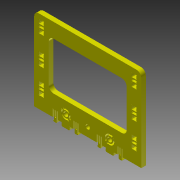
# Autodesk Inventor part: back
Saved by Autodesk Inventor 2012 (Build 160160000, 160)
## iProperties
Created: 2011-10-14
Part Number: back
Document SubType Name: Modeling
Designer: cramera
Density: 0.952 g/cm^3
Material: High Density Polyethylene
Mass: 370.231 g
Surface Area: 1050.09 cm^2
Volume: 388.898 cm^3
Autodesk Inventor part; units mm, degrees
ref_plane "YZ Plane" through (0, 0, 0) normal (1, 0, 0) x (0, 1, 0)
ref_plane "XZ Plane" through (0, 0, 0) normal (0, 1, 0) x (-1, 0, 0)
ref_plane "XY Plane" through (0, 0, 0) normal (0, 0, 1) x (1, 0, 0)
derived "skeleton.ipt"
sketch "POCKET_1-16" plane through (0, 0, 0) normal (0, 0, 1) x (1, 0, 0)
  circle A0 centre (662.3461, 379.1269) radius 7.3978
  constraints: 1 centre point
sketch "STOCK_12MM" plane through (0, 0, 0) normal (0, 0, 1) x (1, 0, 0)
  line L0 (457.2, 914.4) -> (457.2, 0)
  line L1 (457.2, 0) -> (457.2, 914.4)
  line L2 (457.2, 0) -> (914.4, 0)
  line L3 (914.4, 0) -> (914.4, 914.4)
  line L4 (914.4, 914.4) -> (457.2, 914.4)
  constraints: 10 end point
sketch "THROUGH-CUT" plane through (0, 0, 0) normal (0, 0, 1) x (1, 0, 0)
  arc A0 (777.0271, 478.4952) -> (779.2722, 476.2502) centre (778.1496, 477.3727) ccw
  line L0 (777.0271, 478.4952) -> (777.0271, 484.1651)
  arc A1 (779.2722, 486.4102) -> (777.0271, 484.1651) centre (778.1496, 485.2876) ccw
  line L1 (779.2722, 486.4102) -> (787.101, 486.4102)
  arc A2 (789.3461, 486.4102) -> (787.101, 486.4102) centre (788.2236, 485.2876) ccw
  arc A3 (789.3461, 484.1651) -> (789.3461, 486.4102) centre (788.2236, 485.2876) ccw
  line L2 (789.3461, 484.1651) -> (789.3461, 478.4952)
  arc A4 (789.3461, 476.2502) -> (789.3461, 478.4952) centre (788.2236, 477.3727) ccw
  arc A5 (787.101, 476.2502) -> (789.3461, 476.2502) centre (788.2236, 477.3727) ccw
  line L3 (787.101, 476.2502) -> (779.2722, 476.2502)
  line L4 (777.0271, 403.4382) -> (777.0271, 404.0281)
  arc A6 (777.0271, 406.2732) -> (777.0271, 404.0281) centre (778.1496, 405.1506) ccw
  arc A7 (779.2722, 406.2732) -> (777.0271, 406.2732) centre (778.1496, 405.1506) ccw
  line L5 (779.2722, 406.2732) -> (787.101, 406.2732)
  arc A8 (789.3461, 406.2732) -> (787.101, 406.2732) centre (788.2236, 405.1506) ccw
  arc A9 (789.3461, 404.0281) -> (789.3461, 406.2732) centre (788.2236, 405.1506) ccw
  line L6 (789.3461, 404.0281) -> (789.3461, 403.4382)
  arc A10 (787.101, 401.1932) -> (789.3461, 403.4382) centre (788.2236, 402.3157) ccw
  line L7 (787.101, 401.1932) -> (779.2722, 401.1932)
  arc A11 (777.0271, 403.4382) -> (779.2722, 401.1932) centre (778.1496, 402.3157) ccw
  line L8 (547.6651, 543.7281) -> (547.6651, 543.1382)
  arc A12 (547.6651, 540.8932) -> (547.6651, 543.1382) centre (546.5426, 542.0157) ccw
  arc A13 (545.42, 540.8932) -> (547.6651, 540.8932) centre (546.5426, 542.0157) ccw
  line L9 (545.42, 540.8932) -> (537.5912, 540.8932)
  arc A14 (535.3461, 543.1382) -> (537.5912, 540.8932) centre (536.4686, 542.0157) ccw
  line L10 (535.3461, 543.1382) -> (535.3461, 543.7281)
  arc A15 (535.3461, 545.9732) -> (535.3461, 543.7281) centre (536.4686, 544.8506) ccw
  arc A16 (537.5912, 545.9732) -> (535.3461, 545.9732) centre (536.4686, 544.8506) ccw
  line L11 (537.5912, 545.9732) -> (545.42, 545.9732)
  arc A17 (547.6651, 543.7281) -> (545.42, 545.9732) centre (546.5426, 544.8506) ccw
  circle A18 centre (719.4961, 379.1269) radius 5.925
  circle A19 centre (605.1961, 379.1269) radius 5.925
  circle A20 centre (662.3461, 379.1269) radius 5.5563
  line L12 (547.6651, 395.6461) -> (547.6651, 389.9762)
  arc A21 (547.6651, 387.7312) -> (547.6651, 389.9762) centre (546.5426, 388.8537) ccw
  arc A22 (545.42, 387.7312) -> (547.6651, 387.7312) centre (546.5426, 388.8537) ccw
  line L13 (545.42, 387.7312) -> (537.5912, 387.7312)
  arc A23 (535.3461, 389.9762) -> (537.5912, 387.7312) centre (536.4686, 388.8537) ccw
  line L14 (535.3461, 389.9762) -> (535.3461, 395.6461)
  arc A24 (537.5912, 397.8912) -> (535.3461, 395.6461) centre (536.4686, 396.7686) ccw
  line L15 (537.5912, 397.8912) -> (545.42, 397.8912)
  arc A25 (547.6651, 395.6461) -> (545.42, 397.8912) centre (546.5426, 396.7686) ccw
  line L16 (777.0271, 529.6762) -> (777.0271, 535.3461)
  arc A26 (777.0271, 537.5912) -> (777.0271, 535.3461) centre (778.1496, 536.4686) ccw
  arc A27 (779.2722, 537.5912) -> (777.0271, 537.5912) centre (778.1496, 536.4686) ccw
  line L17 (779.2722, 537.5912) -> (787.101, 537.5912)
  arc A28 (789.3461, 537.5912) -> (787.101, 537.5912) centre (788.2236, 536.4686) ccw
  arc A29 (789.3461, 535.3461) -> (789.3461, 537.5912) centre (788.2236, 536.4686) ccw
  line L18 (789.3461, 535.3461) -> (789.3461, 529.6762)
  arc A30 (789.3461, 527.4312) -> (789.3461, 529.6762) centre (788.2236, 528.5537) ccw
  arc A31 (787.101, 527.4312) -> (789.3461, 527.4312) centre (788.2236, 528.5537) ccw
  line L19 (787.101, 527.4312) -> (779.2722, 527.4312)
  arc A32 (777.0271, 529.6762) -> (779.2722, 527.4312) centre (778.1496, 528.5537) ccw
  line L20 (547.6651, 404.0281) -> (547.6651, 403.4382)
  arc A33 (547.6651, 401.1932) -> (547.6651, 403.4382) centre (546.5426, 402.3157) ccw
  arc A34 (545.42, 401.1932) -> (547.6651, 401.1932) centre (546.5426, 402.3157) ccw
  line L21 (545.42, 401.1932) -> (537.5912, 401.1932)
  arc A35 (535.3461, 403.4382) -> (537.5912, 401.1932) centre (536.4686, 402.3157) ccw
  line L22 (535.3461, 403.4382) -> (535.3461, 404.0281)
  arc A36 (537.5912, 406.2732) -> (535.3461, 404.0281) centre (536.4686, 405.1506) ccw
  line L23 (537.5912, 406.2732) -> (545.42, 406.2732)
  arc A37 (547.6651, 406.2732) -> (545.42, 406.2732) centre (546.5426, 405.1506) ccw
  arc A38 (547.6651, 404.0281) -> (547.6651, 406.2732) centre (546.5426, 405.1506) ccw
  line L24 (779.2722, 559.4352) -> (787.101, 559.4352)
  arc A39 (789.3461, 559.4352) -> (787.101, 559.4352) centre (788.2236, 558.3126) ccw
  arc A40 (789.3461, 557.1901) -> (789.3461, 559.4352) centre (788.2236, 558.3126) ccw
  line L25 (789.3461, 557.1901) -> (789.3461, 551.5202)
  arc A41 (789.3461, 549.2752) -> (789.3461, 551.5202) centre (788.2236, 550.3977) ccw
  arc A42 (787.101, 549.2752) -> (789.3461, 549.2752) centre (788.2236, 550.3977) ccw
  line L26 (787.101, 549.2752) -> (779.2722, 549.2752)
  arc A43 (777.0271, 549.2752) -> (779.2722, 549.2752) centre (778.1496, 550.3977) ccw
  arc A44 (777.0271, 551.5202) -> (777.0271, 549.2752) centre (778.1496, 550.3977) ccw
  line L27 (777.0271, 551.5202) -> (777.0271, 557.1901)
  arc A45 (779.2722, 559.4352) -> (777.0271, 557.1901) centre (778.1496, 558.3126) ccw
  arc A46 (779.2722, 419.7352) -> (777.0271, 417.4901) centre (778.1496, 418.6126) ccw
  line L28 (779.2722, 419.7352) -> (787.101, 419.7352)
  arc A47 (789.3461, 419.7352) -> (787.101, 419.7352) centre (788.2236, 418.6126) ccw
  arc A48 (789.3461, 417.4901) -> (789.3461, 419.7352) centre (788.2236, 418.6126) ccw
  line L29 (789.3461, 417.4901) -> (789.3461, 411.8202)
  arc A49 (789.3461, 409.5752) -> (789.3461, 411.8202) centre (788.2236, 410.6977) ccw
  arc A50 (787.101, 409.5752) -> (789.3461, 409.5752) centre (788.2236, 410.6977) ccw
  line L30 (787.101, 409.5752) -> (779.2722, 409.5752)
  arc A51 (777.0271, 411.8202) -> (779.2722, 409.5752) centre (778.1496, 410.6977) ccw
  line L31 (777.0271, 411.8202) -> (777.0271, 417.4901)
  arc A52 (777.0271, 456.6512) -> (779.2722, 454.4062) centre (778.1496, 455.5287) ccw
  line L32 (777.0271, 456.6512) -> (777.0271, 462.3211)
  arc A53 (779.2722, 464.5662) -> (777.0271, 462.3211) centre (778.1496, 463.4436) ccw
  line L33 (779.2722, 464.5662) -> (787.101, 464.5662)
  arc A54 (789.3461, 464.5662) -> (787.101, 464.5662) centre (788.2236, 463.4436) ccw
  arc A55 (789.3461, 462.3211) -> (789.3461, 464.5662) centre (788.2236, 463.4436) ccw
  line L34 (789.3461, 462.3211) -> (789.3461, 456.6512)
  arc A56 (789.3461, 454.4062) -> (789.3461, 456.6512) centre (788.2236, 455.5287) ccw
  arc A57 (787.101, 454.4062) -> (789.3461, 454.4062) centre (788.2236, 455.5287) ccw
  line L35 (787.101, 454.4062) -> (779.2722, 454.4062)
  arc A58 (777.0271, 389.9762) -> (777.0271, 387.7312) centre (778.1496, 388.8537) ccw
  line L36 (777.0271, 389.9762) -> (777.0271, 395.6461)
  arc A59 (779.2722, 397.8912) -> (777.0271, 395.6461) centre (778.1496, 396.7686) ccw
  line L37 (779.2722, 397.8912) -> (787.101, 397.8912)
  arc A60 (789.3461, 397.8912) -> (787.101, 397.8912) centre (788.2236, 396.7686) ccw
  arc A61 (789.3461, 395.6461) -> (789.3461, 397.8912) centre (788.2236, 396.7686) ccw
  line L38 (789.3461, 395.6461) -> (789.3461, 389.9762)
  arc A62 (787.101, 387.7312) -> (789.3461, 389.9762) centre (788.2236, 388.8537) ccw
  line L39 (787.101, 387.7312) -> (779.2722, 387.7312)
  arc A63 (777.0271, 387.7312) -> (779.2722, 387.7312) centre (778.1496, 388.8537) ccw
  line L40 (547.6651, 484.1651) -> (547.6651, 478.4952)
  arc A64 (547.6651, 476.2502) -> (547.6651, 478.4952) centre (546.5426, 477.3727) ccw
  arc A65 (545.42, 476.2502) -> (547.6651, 476.2502) centre (546.5426, 477.3727) ccw
  line L41 (545.42, 476.2502) -> (537.5912, 476.2502)
  arc A66 (535.3461, 478.4952) -> (537.5912, 476.2502) centre (536.4686, 477.3727) ccw
  line L42 (535.3461, 478.4952) -> (535.3461, 484.1651)
  arc A67 (537.5912, 486.4102) -> (535.3461, 484.1651) centre (536.4686, 485.2876) ccw
  line L43 (537.5912, 486.4102) -> (545.42, 486.4102)
  arc A68 (547.6651, 484.1651) -> (545.42, 486.4102) centre (546.5426, 485.2876) ccw
  arc A69 (777.0271, 543.1382) -> (777.0271, 540.8932) centre (778.1496, 542.0157) ccw
  line L44 (777.0271, 543.1382) -> (777.0271, 543.7281)
  arc A70 (779.2722, 545.9732) -> (777.0271, 543.7281) centre (778.1496, 544.8506) ccw
  line L45 (779.2722, 545.9732) -> (787.101, 545.9732)
  arc A71 (789.3461, 545.9732) -> (787.101, 545.9732) centre (788.2236, 544.8506) ccw
  arc A72 (789.3461, 543.7281) -> (789.3461, 545.9732) centre (788.2236, 544.8506) ccw
  line L46 (789.3461, 543.7281) -> (789.3461, 543.1382)
  arc A73 (789.3461, 540.8932) -> (789.3461, 543.1382) centre (788.2236, 542.0157) ccw
  arc A74 (787.101, 540.8932) -> (789.3461, 540.8932) centre (788.2236, 542.0157) ccw
  line L47 (787.101, 540.8932) -> (779.2722, 540.8932)
  arc A75 (777.0271, 540.8932) -> (779.2722, 540.8932) centre (778.1496, 542.0157) ccw
  line L48 (547.6651, 470.7031) -> (547.6651, 470.1132)
  arc A76 (547.6651, 467.8682) -> (547.6651, 470.1132) centre (546.5426, 468.9907) ccw
  arc A77 (545.42, 467.8682) -> (547.6651, 467.8682) centre (546.5426, 468.9907) ccw
  line L49 (545.42, 467.8682) -> (537.5912, 467.8682)
  arc A78 (535.3461, 470.1132) -> (537.5912, 467.8682) centre (536.4686, 468.9907) ccw
  line L50 (535.3461, 470.1132) -> (535.3461, 470.7031)
  arc A79 (537.5912, 472.9482) -> (535.3461, 470.7031) centre (536.4686, 471.8256) ccw
  line L51 (537.5912, 472.9482) -> (545.42, 472.9482)
  arc A80 (547.6651, 470.7031) -> (545.42, 472.9482) centre (546.5426, 471.8256) ccw
  line L52 (547.6651, 417.4901) -> (547.6651, 411.8202)
  arc A81 (547.6651, 409.5752) -> (547.6651, 411.8202) centre (546.5426, 410.6977) ccw
  arc A82 (545.42, 409.5752) -> (547.6651, 409.5752) centre (546.5426, 410.6977) ccw
  line L53 (545.42, 409.5752) -> (537.5912, 409.5752)
  arc A83 (535.3461, 411.8202) -> (537.5912, 409.5752) centre (536.4686, 410.6977) ccw
  line L54 (535.3461, 411.8202) -> (535.3461, 417.4901)
  arc A84 (537.5912, 419.7352) -> (535.3461, 417.4901) centre (536.4686, 418.6126) ccw
  line L55 (537.5912, 419.7352) -> (545.42, 419.7352)
  arc A85 (547.6651, 417.4901) -> (545.42, 419.7352) centre (546.5426, 418.6126) ccw
  line L56 (547.6651, 557.1901) -> (547.6651, 551.5202)
  arc A86 (547.6651, 549.2752) -> (547.6651, 551.5202) centre (546.5426, 550.3977) ccw
  arc A87 (545.42, 549.2752) -> (547.6651, 549.2752) centre (546.5426, 550.3977) ccw
  line L57 (545.42, 549.2752) -> (537.5912, 549.2752)
  arc A88 (535.3461, 551.5202) -> (537.5912, 549.2752) centre (536.4686, 550.3977) ccw
  line L58 (535.3461, 551.5202) -> (535.3461, 557.1901)
  arc A89 (537.5912, 559.4352) -> (535.3461, 557.1901) centre (536.4686, 558.3126) ccw
  line L59 (537.5912, 559.4352) -> (545.42, 559.4352)
  arc A90 (547.6651, 557.1901) -> (545.42, 559.4352) centre (546.5426, 558.3126) ccw
  line L60 (535.3461, 456.6512) -> (535.3461, 462.3211)
  arc A91 (537.5912, 464.5662) -> (535.3461, 462.3211) centre (536.4686, 463.4436) ccw
  line L61 (537.5912, 464.5662) -> (545.42, 464.5662)
  arc A92 (547.6651, 462.3211) -> (545.42, 464.5662) centre (546.5426, 463.4436) ccw
  line L62 (547.6651, 462.3211) -> (547.6651, 456.6512)
  arc A93 (545.42, 454.4062) -> (547.6651, 456.6512) centre (546.5426, 455.5287) ccw
  line L63 (545.42, 454.4062) -> (537.5912, 454.4062)
  arc A94 (535.3461, 456.6512) -> (537.5912, 454.4062) centre (536.4686, 455.5287) ccw
  arc A95 (777.0271, 470.1132) -> (777.0271, 467.8682) centre (778.1496, 468.9907) ccw
  line L64 (777.0271, 470.1132) -> (777.0271, 470.7031)
  arc A96 (779.2722, 472.9482) -> (777.0271, 470.7031) centre (778.1496, 471.8256) ccw
  line L65 (779.2722, 472.9482) -> (787.101, 472.9482)
  arc A97 (789.3461, 472.9482) -> (787.101, 472.9482) centre (788.2236, 471.8256) ccw
  arc A98 (789.3461, 470.7031) -> (789.3461, 472.9482) centre (788.2236, 471.8256) ccw
  line L66 (789.3461, 470.7031) -> (789.3461, 470.1132)
  arc A99 (787.101, 467.8682) -> (789.3461, 470.1132) centre (788.2236, 468.9907) ccw
  line L67 (787.101, 467.8682) -> (779.2722, 467.8682)
  arc A100 (777.0271, 467.8682) -> (779.2722, 467.8682) centre (778.1496, 468.9907) ccw
  line L68 (535.3461, 529.6762) -> (535.3461, 535.3461)
  arc A101 (537.5912, 537.5912) -> (535.3461, 535.3461) centre (536.4686, 536.4686) ccw
  line L69 (537.5912, 537.5912) -> (545.42, 537.5912)
  arc A102 (547.6651, 535.3461) -> (545.42, 537.5912) centre (546.5426, 536.4686) ccw
  line L70 (547.6651, 535.3461) -> (547.6651, 529.6762)
  arc A103 (545.42, 527.4312) -> (547.6651, 529.6762) centre (546.5426, 528.5537) ccw
  line L71 (545.42, 527.4312) -> (537.5912, 527.4312)
  arc A104 (535.3461, 529.6762) -> (537.5912, 527.4312) centre (536.4686, 528.5537) ccw
  arc A105 (723.7603, 390.4675) -> (708.1555, 374.8628) centre (719.4961, 379.1269) ccw
  line L72 (708.1555, 374.8628) -> (707.4839, 374.1911)
  arc A106 (707.4839, 374.1911) -> (707.4839, 371.9461) centre (708.6064, 373.0686) ccw
  line L73 (707.4839, 371.9461) -> (707.5557, 371.8742)
  arc A107 (707.5557, 371.8742) -> (709.8008, 371.8742) centre (708.6782, 372.9968) ccw
  line L74 (709.8008, 371.8742) -> (711.2845, 373.3579)
  arc A108 (711.2845, 373.3579) -> (711.5831, 375.1879) centre (710.1619, 374.4805) ccw
  arc A109 (723.4351, 387.0399) -> (711.5831, 375.1879) centre (719.4961, 379.1269) ccw
  arc A110 (723.4351, 387.0399) -> (725.2651, 387.3385) centre (724.1426, 388.4611) ccw
  line L75 (725.2651, 387.3385) -> (726.7488, 388.8223)
  arc A111 (726.7488, 388.8223) -> (726.7488, 391.0673) centre (725.6263, 389.9448) ccw
  line L76 (726.7488, 391.0673) -> (726.677, 391.1392)
  arc A112 (726.677, 391.1392) -> (724.4319, 391.1392) centre (725.5544, 390.0166) ccw
  line L77 (724.4319, 391.1392) -> (723.7603, 390.4675)
  line L78 (763.9461, 521.2082) -> (763.9461, 422.7832)
  arc A113 (751.2461, 410.0832) -> (763.9461, 422.7832) centre (751.2461, 422.7832) ccw
  line L79 (751.2461, 410.0832) -> (573.4461, 410.0832)
  arc A114 (560.7461, 422.7832) -> (573.4461, 410.0832) centre (573.4461, 422.7832) ccw
  line L80 (560.7461, 422.7832) -> (560.7461, 521.2082)
  arc A115 (573.4461, 533.9082) -> (560.7461, 521.2082) centre (573.4461, 521.2082) ccw
  line L81 (573.4461, 533.9082) -> (751.2461, 533.9082)
  arc A116 (763.9461, 521.2082) -> (751.2461, 533.9082) centre (751.2461, 521.2082) ccw
  arc A117 (577.9048, 357.2797) -> (579.4923, 358.8672) centre (577.9048, 358.8672) ccw
  line L82 (577.9048, 357.2797) -> (577.7778, 357.2797)
  arc A118 (576.1903, 358.8672) -> (577.7778, 357.2797) centre (577.7778, 358.8672) ccw
  line L83 (576.1903, 358.8672) -> (576.1903, 373.5707)
  arc A119 (577.7778, 375.1582) -> (576.1903, 373.5707) centre (577.7778, 373.5707) ccw
  line L84 (577.7778, 375.1582) -> (577.9048, 375.1582)
  arc A120 (579.4923, 373.5707) -> (577.9048, 375.1582) centre (577.9048, 373.5707) ccw
  line L85 (579.4923, 373.5707) -> (579.4923, 358.8672)
  arc A121 (692.6854, 357.2797) -> (694.2729, 358.8672) centre (692.6854, 358.8672) ccw
  line L86 (692.6854, 357.2797) -> (692.5584, 357.2797)
  arc A122 (690.9709, 358.8672) -> (692.5584, 357.2797) centre (692.5584, 358.8672) ccw
  line L87 (690.9709, 358.8672) -> (690.9709, 373.5707)
  arc A123 (692.5584, 375.1582) -> (690.9709, 373.5707) centre (692.5584, 373.5707) ccw
  line L88 (692.5584, 375.1582) -> (692.6732, 375.1582)
  arc A124 (694.2607, 373.5707) -> (692.6732, 375.1582) centre (692.6732, 373.5707) ccw
  line L89 (694.2607, 373.5707) -> (694.2729, 358.8672)
  arc A125 (745.1999, 358.8672) -> (746.7874, 357.2797) centre (746.7874, 358.8672) ccw
  line L90 (746.7874, 357.2797) -> (746.9144, 357.2797)
  arc A126 (746.9144, 357.2797) -> (748.5019, 358.8672) centre (746.9144, 358.8672) ccw
  line L91 (748.5019, 358.8672) -> (748.5019, 373.5707)
  arc A127 (748.5019, 373.5707) -> (746.9144, 375.1582) centre (746.9144, 373.5707) ccw
  line L92 (746.9144, 375.1582) -> (746.7874, 375.1582)
  arc A128 (746.7874, 375.1582) -> (745.1999, 373.5707) centre (746.7874, 373.5707) ccw
  line L93 (745.1999, 373.5707) -> (745.1999, 358.8672)
  arc A129 (632.1338, 357.2797) -> (633.7213, 358.8672) centre (632.1338, 358.8672) ccw
  line L94 (633.7213, 358.8672) -> (633.7213, 373.5707)
  arc A130 (633.7213, 373.5707) -> (632.1338, 375.1582) centre (632.1338, 373.5707) ccw
  line L95 (632.1338, 375.1582) -> (632.0068, 375.1582)
  arc A131 (632.0068, 375.1582) -> (630.4193, 373.5707) centre (632.0068, 373.5707) ccw
  line L96 (630.4193, 373.5707) -> (630.4193, 358.8672)
  arc A132 (630.4193, 358.8672) -> (632.0068, 357.2797) centre (632.0068, 358.8672) ccw
  line L97 (632.0068, 357.2797) -> (632.1338, 357.2797)
  arc A133 (593.1839, 386.3078) -> (593.1839, 384.0627) centre (594.3064, 385.1853) ccw
  line L98 (593.1839, 384.0627) -> (593.8555, 383.3911)
  arc A134 (593.8555, 383.3911) -> (609.4603, 367.7863) centre (605.1961, 379.1269) ccw
  line L99 (609.4603, 367.7863) -> (610.1319, 367.1147)
  arc A135 (610.1319, 367.1147) -> (612.377, 367.1147) centre (611.2544, 368.2372) ccw
  line L100 (612.377, 367.1147) -> (612.4488, 367.1865)
  arc A136 (612.4488, 367.1865) -> (612.4488, 369.4316) centre (611.3263, 368.3091) ccw
  line L101 (612.4488, 369.4316) -> (610.9651, 370.9153)
  arc A137 (610.9651, 370.9153) -> (609.1351, 371.2139) centre (609.8426, 369.7928) ccw
  arc A138 (597.2831, 383.0659) -> (609.1351, 371.2139) centre (605.1961, 379.1269) ccw
  arc A139 (597.2831, 383.0659) -> (596.9845, 384.8959) centre (595.8619, 383.7734) ccw
  line L102 (596.9845, 384.8959) -> (595.5008, 386.3796)
  arc A140 (595.5008, 386.3796) -> (593.2557, 386.3796) centre (594.3782, 385.2571) ccw
  line L103 (593.2557, 386.3796) -> (593.1839, 386.3078)
  arc A141 (617.2083, 371.9461) -> (617.2083, 374.1911) centre (616.0858, 373.0686) ccw
  line L104 (617.2083, 374.1911) -> (616.5367, 374.8628)
  arc A142 (616.5367, 374.8628) -> (600.9319, 390.4675) centre (605.1961, 379.1269) ccw
  line L105 (600.9319, 390.4675) -> (600.2603, 391.1392)
  arc A143 (600.2603, 391.1392) -> (598.0152, 391.1392) centre (599.1378, 390.0166) ccw
  line L106 (598.0152, 391.1392) -> (597.9434, 391.0673)
  arc A144 (597.9434, 391.0673) -> (597.9434, 388.8223) centre (599.0659, 389.9448) ccw
  line L107 (597.9434, 388.8223) -> (599.4271, 387.3385)
  arc A145 (599.4271, 387.3385) -> (601.2571, 387.0399) centre (600.5496, 388.4611) ccw
  arc A146 (613.1091, 375.1879) -> (601.2571, 387.0399) centre (605.1961, 379.1269) ccw
  arc A147 (613.1091, 375.1879) -> (613.4077, 373.3579) centre (614.5302, 374.4805) ccw
  line L108 (613.4077, 373.3579) -> (614.8914, 371.8742)
  arc A148 (614.8914, 371.8742) -> (617.1365, 371.8742) centre (616.014, 372.9968) ccw
  line L109 (617.1365, 371.8742) -> (617.2083, 371.9461)
  line L110 (629.9748, 347.2182) -> (633.6777, 347.2182)
  line L111 (633.6777, 347.2182) -> (637.2773, 348.0403)
  line L112 (637.2773, 348.0403) -> (637.2773, 349.7582)
  line L113 (637.2773, 349.7582) -> (635.7533, 351.0282)
  line L114 (635.7533, 351.0282) -> (635.7533, 353.6554)
  line L115 (635.7533, 353.6554) -> (635.7533, 373.5707)
  arc A149 (637.3408, 375.1582) -> (635.7533, 373.5707) centre (637.3408, 373.5707) ccw
  line L116 (637.3408, 375.1582) -> (637.4678, 375.1582)
  arc A150 (639.0553, 373.5707) -> (637.4678, 375.1582) centre (637.4678, 373.5707) ccw
  line L117 (639.0553, 373.5707) -> (639.0553, 356.1082)
  line L118 (639.0553, 356.1082) -> (685.6369, 356.1082)
  line L119 (685.6369, 356.1082) -> (685.6369, 373.5707)
  arc A151 (687.2244, 375.1582) -> (685.6369, 373.5707) centre (687.2244, 373.5707) ccw
  line L120 (687.2244, 375.1582) -> (687.3514, 375.1582)
  arc A152 (688.9389, 373.5707) -> (687.3514, 375.1582) centre (687.3514, 373.5707) ccw
  line L121 (688.9389, 373.5707) -> (688.9389, 353.6554)
  line L122 (688.9389, 353.6554) -> (688.9389, 351.0282)
  line L123 (688.9389, 351.0282) -> (687.4149, 349.7582)
  line L124 (687.4149, 349.7582) -> (687.4149, 348.0403)
  line L125 (687.4149, 348.0403) -> (691.0145, 347.2182)
  line L126 (691.0145, 347.2182) -> (694.7174, 347.2182)
  arc A153 (694.7174, 347.2182) -> (696.3049, 348.8057) centre (694.7174, 348.8057) ccw
  line L127 (696.3049, 348.8057) -> (696.3049, 373.5707)
  arc A154 (697.8924, 375.1582) -> (696.3049, 373.5707) centre (697.8924, 373.5707) ccw
  line L128 (697.8924, 375.1582) -> (698.0194, 375.1582)
  arc A155 (699.6069, 373.5707) -> (698.0194, 375.1582) centre (698.0194, 373.5707) ccw
  line L129 (699.6069, 373.5707) -> (699.6069, 356.1082)
  line L130 (699.6069, 356.1082) -> (707.0139, 356.1082)
  arc A156 (709.2589, 353.8631) -> (707.0139, 356.1082) centre (708.1364, 354.9856) ccw
  line L131 (709.2589, 353.8631) -> (709.2589, 348.8057)
  line L132 (709.2589, 348.8057) -> (710.8464, 347.2182)
  line L133 (710.8464, 347.2182) -> (728.6264, 347.2182)
  line L134 (728.6264, 347.2182) -> (730.2139, 348.8057)
  line L135 (730.2139, 348.8057) -> (730.2139, 353.8631)
  arc A157 (732.459, 356.1082) -> (730.2139, 353.8631) centre (731.3364, 354.9856) ccw
  line L136 (732.459, 356.1082) -> (739.8659, 356.1082)
  line L137 (739.8659, 356.1082) -> (739.8659, 373.5707)
  arc A158 (741.4534, 375.1582) -> (739.8659, 373.5707) centre (741.4534, 373.5707) ccw
  line L138 (741.4534, 375.1582) -> (741.5804, 375.1582)
  arc A159 (743.1679, 373.5707) -> (741.5804, 375.1582) centre (741.5804, 373.5707) ccw
  line L139 (743.1679, 373.5707) -> (743.1679, 348.8057)
  arc A160 (743.1679, 348.8057) -> (744.7532, 347.2182) centre (744.7554, 348.8057) ccw
  line L140 (744.7532, 347.2182) -> (748.4584, 347.2182)
  line L141 (748.4584, 347.2182) -> (752.0579, 348.0403)
  line L142 (752.0579, 348.0403) -> (752.0579, 349.7582)
  line L143 (752.0579, 349.7582) -> (750.5339, 351.0282)
  line L144 (750.5339, 351.0282) -> (750.5339, 353.6554)
  line L145 (750.5339, 353.6554) -> (750.5339, 373.5707)
  arc A161 (752.1214, 375.1582) -> (750.5339, 373.5707) centre (752.1214, 373.5707) ccw
  line L146 (752.1214, 375.1582) -> (752.2484, 375.1582)
  arc A162 (753.8359, 373.5707) -> (752.2484, 375.1582) centre (752.2484, 373.5707) ccw
  line L147 (753.8359, 373.5707) -> (753.8359, 356.1082)
  line L148 (753.8359, 356.1082) -> (802.0461, 356.1082)
  line L149 (802.0461, 356.1082) -> (802.0461, 559.3082)
  arc A163 (802.0461, 559.3082) -> (789.3461, 572.0082) centre (789.3461, 559.3082) ccw
  line L150 (789.3461, 572.0082) -> (535.3461, 572.0082)
  arc A164 (535.3461, 572.0082) -> (522.6461, 559.3082) centre (535.3461, 559.3082) ccw
  line L151 (522.6461, 559.3082) -> (522.6461, 356.1082)
  line L152 (522.6461, 356.1082) -> (570.8563, 356.1082)
  line L153 (570.8563, 356.1082) -> (570.8563, 373.5707)
  arc A165 (572.4438, 375.1582) -> (570.8563, 373.5707) centre (572.4438, 373.5707) ccw
  line L154 (572.4438, 375.1582) -> (572.5708, 375.1582)
  arc A166 (574.1583, 373.5707) -> (572.5708, 375.1582) centre (572.5708, 373.5707) ccw
  line L155 (574.1583, 373.5707) -> (574.1583, 353.6554)
  line L156 (574.1583, 353.6554) -> (574.1583, 351.0282)
  line L157 (574.1583, 351.0282) -> (572.6343, 349.7582)
  line L158 (572.6343, 349.7582) -> (572.6343, 348.0403)
  line L159 (572.6343, 348.0403) -> (576.2338, 347.2182)
  line L160 (576.2338, 347.2182) -> (579.9389, 347.2182)
  arc A167 (579.9389, 347.2182) -> (581.5243, 348.8057) centre (579.9368, 348.8057) ccw
  line L161 (581.5243, 348.8057) -> (581.5243, 373.5707)
  arc A168 (583.1118, 375.1582) -> (581.5243, 373.5707) centre (583.1118, 373.5707) ccw
  line L162 (583.1118, 375.1582) -> (583.2388, 375.1582)
  arc A169 (584.8263, 373.5707) -> (583.2388, 375.1582) centre (583.2388, 373.5707) ccw
  line L163 (584.8263, 373.5707) -> (584.8263, 356.1082)
  line L164 (584.8263, 356.1082) -> (592.2332, 356.1082)
  arc A170 (594.4783, 353.8631) -> (592.2332, 356.1082) centre (593.3557, 354.9856) ccw
  line L165 (594.4783, 353.8631) -> (594.4783, 348.8057)
  line L166 (594.4783, 348.8057) -> (596.0658, 347.2182)
  line L167 (596.0658, 347.2182) -> (613.8458, 347.2182)
  line L168 (613.8458, 347.2182) -> (615.4333, 348.8057)
  line L169 (615.4333, 348.8057) -> (615.4333, 353.8631)
  arc A171 (617.6783, 356.1082) -> (615.4333, 353.8631) centre (616.5558, 354.9856) ccw
  line L170 (617.6783, 356.1082) -> (625.0853, 356.1082)
  line L171 (625.0853, 356.1082) -> (625.0853, 373.5707)
  arc A172 (626.6728, 375.1582) -> (625.0853, 373.5707) centre (626.6728, 373.5707) ccw
  line L172 (626.6728, 375.1582) -> (626.7998, 375.1582)
  arc A173 (628.3873, 373.5707) -> (626.7998, 375.1582) centre (626.7998, 373.5707) ccw
  line L173 (628.3873, 373.5707) -> (628.3873, 348.8057)
  arc A174 (628.3873, 348.8057) -> (629.9748, 347.2182) centre (629.9748, 348.8057) ccw
  arc A175 (712.3152, 367.1147) -> (714.5603, 367.1147) centre (713.4378, 368.2372) ccw
  line L174 (714.5603, 367.1147) -> (715.2319, 367.7863)
  arc A176 (715.2319, 367.7863) -> (730.8367, 383.3911) centre (719.4961, 379.1269) ccw
  line L175 (730.8367, 383.3911) -> (731.5083, 384.0627)
  arc A177 (731.5083, 384.0627) -> (731.5083, 386.3078) centre (730.3858, 385.1853) ccw
  line L176 (731.5083, 386.3078) -> (731.4365, 386.3796)
  arc A178 (731.4365, 386.3796) -> (729.1867, 386.3749) centre (730.3139, 385.2571) ccw
  line L177 (729.1867, 386.3749) -> (727.7077, 384.8959)
  arc A179 (727.7077, 384.8959) -> (727.4091, 383.0659) centre (728.8302, 383.7734) ccw
  arc A180 (715.5571, 371.2139) -> (727.4091, 383.0659) centre (719.4961, 379.1269) ccw
  arc A181 (715.5571, 371.2139) -> (713.7271, 370.9153) centre (714.8496, 369.7928) ccw
  line L178 (713.7271, 370.9153) -> (712.2434, 369.4316)
  arc A182 (712.2434, 369.4316) -> (712.2434, 367.1865) centre (713.3659, 368.3091) ccw
  line L179 (712.2434, 367.1865) -> (712.3152, 367.1147)
  dimension "d5" = 11.85
  dimension "d6" = 11.85
  constraints: 360 end point, 360 point on circle, 183 centre point
  measures "d5" diameter of A19
  measures "d6" diameter of A18
extrude "Extrusion1" add sketch "THROUGH-CUT" along normal blind 12
extrude "Extrusion2" cut sketch "POCKET_1-16" along normal blind 1.5875
equation "\"d6\" = d5"
equation "\"d1\" = StockThickness"
equation "\"StockThickness\" = 12"
body "Solid1"
